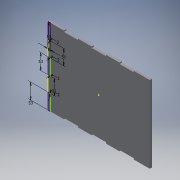
# Autodesk Inventor part: BASE
Saved by Autodesk Inventor 2016 (Build 200138000, 138)
## iProperties
Created: 2017-06-07
Part Number: BASE
Material: Generic
Document SubType Name: Modeling
Designer: fabio-note
Density: 1 g/cm^3
Appearance: Default
Author: fabio-note
Autodesk Inventor part; units mm, degrees
ref_plane "YZ Plane" through (0, 0, 0) normal (1, 0, 0) x (0, 1, 0)
ref_plane "XZ Plane" through (0, 0, 0) normal (0, 1, 0) x (-1, 0, 0)
ref_plane "XY Plane" through (0, 0, 0) normal (0, 0, 1) x (1, 0, 0)
sketch "Sketch1" plane through (0, 0, 0) normal (0, 1, 0) x (-1, 0, 0)
  line L0 (173, -130.5) -> (-173, -130.5)
  line L1 (-173, -130.5) -> (-173, 130.5)
  line L2 (-173, 130.5) -> (173, 130.5)
  line L3 (173, 130.5) -> (173, -130.5)
  point P0 (0, 0)
  point P1 (173, 0)
  point P2 (0, -130.5)
  dimension "d0" = 346
  dimension "d1" = 261
  constraints: 8 end point, 2 midpoint, 2 parallel, 1 horizontal, 1 horizontal alignment, 1 perpendicular, 1 vertical alignment
  measures "d0" distance of L1.end L2.end
  measures "d1" distance between parallel lines of L2 L0
extrude "Extrusion1" add sketch "Sketch1" along normal blind 8
sketch "Esboço2" plane through (0, 8, 0) normal (0, 1, 0) x (1, 0, 0)
  line L0 (173, 130.5) -> (-173, 130.5) projected
  line L1 (-118.5, 130.5) -> (-70.5, 130.5)
  line L2 (-70.5, 130.5) -> (-70.5, 126.5)
  line L3 (-70.5, 126.5) -> (-118.5, 126.5)
  line L4 (-118.5, 126.5) -> (-118.5, 130.5)
  line L5 (-173, 130.5) -> (-173, -130.5) projected
  line L6 (-24, 130.5) -> (24, 130.5)
  line L7 (24, 130.5) -> (24, 126.5)
  line L8 (24, 126.5) -> (-24, 126.5)
  line L9 (-24, 126.5) -> (-24, 130.5)
  line L10 (70.5, 130.5) -> (118.5, 130.5)
  line L11 (118.5, 130.5) -> (118.5, 126.5)
  line L12 (118.5, 126.5) -> (70.5, 126.5)
  line L13 (70.5, 126.5) -> (70.5, 130.5)
  line L14 (173, -130.5) -> (173, 130.5) projected
  circle A0 centre (-118.5, 126.5) radius 1
  circle A1 centre (-70.5, 126.5) radius 1
  circle A2 centre (-24, 126.5) radius 1
  circle A3 centre (24, 126.5) radius 1
  circle A4 centre (70.5, 126.5) radius 1
  circle A5 centre (118.5, 126.5) radius 1
  point P0 (0, 0)
  dimension "d4" = 48
  dimension "d5" = 4
  dimension "d6" = 54.5
  dimension "d7" = 48
  dimension "d8" = 4
  dimension "d9" = 46.5
  dimension "d10" = 4
  dimension "d11" = 48
  dimension "d12" = 46.5
  dimension "d13" = 54.5
  dimension "d14" = 2
  dimension "d15" = 2
  dimension "d16" = 2
  dimension "d17" = 2
  constraints: 24 end point, 6 centre point, 6 coincident, 6 parallel, 3 horizontal, 3 perpendicular, 3 point on line
  measures "d4" distance of L2.end L3.end
  measures "d5" distance of L1.end L2.end
  measures "d6" distance between parallel lines of L5 L4
  measures "d7" distance of L7.end L8.end
  measures "d8" distance between parallel lines of L0 L8
  measures "d9" distance between parallel lines of L2 L9
  measures "d10" distance between parallel lines of L12 L10
  measures "d11" distance from line of L12.end L11
  measures "d12" distance from line of L7 L10.start
  measures "d13" distance between parallel lines of L14 L11
  measures "d14" diameter of A0
  measures "d15" diameter of A2
  measures "d16" diameter of A3
  measures "d17" diameter of A4
extrude "Extrusão2" cut sketch "Esboço2" against normal blind 10
mirror "Espelhamento1" about plane through (0, 0, 0) normal (0, 0, 1) of "Extrusão2"
sketch "Esboço3" plane through (0, 0, 0) normal (0, -1, 0) x (1, 0, 0)
  line L0 (-173, 130.5) -> (-173, -130.5) projected
  line L1 (-173, 130.5) -> (-165, 130.5)
  line L2 (-165, 130.5) -> (-165, 77.5)
  line L3 (-165, 77.5) -> (-173, 77.5)
  line L4 (-173, 77.5) -> (-173, 130.5)
  line L5 (-165, 26.5) -> (-173, 26.5)
  line L6 (-173, 26.5) -> (-173, -26.5)
  line L7 (-173, -26.5) -> (-165, -26.5)
  line L8 (-165, -26.5) -> (-165, 26.5)
  line L9 (-173, -130.5) -> (-165, -130.5)
  line L10 (-165, -130.5) -> (-165, -77.5)
  line L11 (-165, -77.5) -> (-173, -77.5)
  line L12 (-173, -77.5) -> (-173, -130.5)
  circle A0 centre (-165, 77.5) radius 1
  circle A1 centre (-165, 26.5) radius 1
  circle A2 centre (-165, -26.5) radius 1
  circle A3 centre (-165, -77.5) radius 1
  point P0 (0, 0)
  dimension "d20" = 8
  dimension "d21" = 53
  dimension "d22" = 53
  dimension "d23" = 51
  dimension "d24" = 51
  dimension "d25" = 53
  dimension "d26" = 2
  dimension "d27" = 2
  dimension "d28" = 2
  dimension "d29" = 2
  constraints: 24 end point, 6 parallel, 4 centre point, 4 coincident, 3 horizontal, 3 perpendicular, 2 point on line
  measures "d20" distance of L2.end L3.end
  measures "d21" distance between parallel lines of L3 L1
  measures "d22" distance of L6.end L5.end
  measures "d23" distance between parallel lines of L3 L5
  measures "d24" distance between parallel lines of L11 L7
  measures "d25" distance from line of L9.start L11
  measures "d26" diameter of A0
  measures "d27" diameter of A1
  measures "d28" diameter of A2
  measures "d29" diameter of A3
extrude "Extrusão3" cut sketch "Esboço3" against normal blind 10
mirror "Espelhamento2" about plane through (0, 0, 0) normal (1, 0, 0) of "Extrusão3"
body "Solid1"
